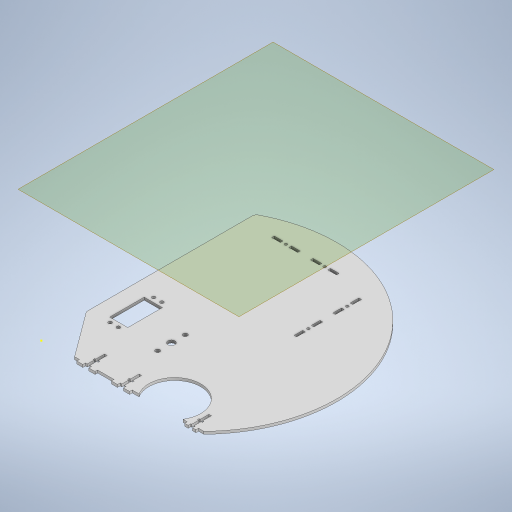
# Autodesk Inventor part: боковые стороны головы
Saved by Autodesk Inventor 2023.2 (Build 272271030, 271C)
## iProperties
Created: 2024-01-31
Part Number: боковые стороны головы
Material: Типовые
Document SubType Name: Modeling
Designer: I9232
Density: 1 g/cm^3
Appearance: По умолчанию
Mass: 147.227 g
Surface Area: 1032.77 cm^2
Volume: 147.227 cm^3
Author: I9232
Autodesk Inventor part; units mm, degrees
ref_plane "YZ Plane" through (0, 0, 0) normal (1, 0, 0) x (0, 1, 0)
ref_plane "XZ Plane" through (0, 0, 0) normal (0, 1, 0) x (-1, 0, 0)
ref_plane "XY Plane" through (0, 0, 0) normal (0, 0, 1) x (1, 0, 0)
sketch "Эскиз1" plane through (0, 0, 0) normal (0, 1, 0) x (-1, 0, 0)
  line L0 (-188.1037, -96.7538) -> (-38.405, -96.7538)
  line L1 (0, -148.7467) -> (0, -343.7987)
  line L2 (-38.405, -96.7538) -> (0, -148.7467)
  arc A0 (-188.1037, -96.7538) -> (0, -343.7987) centre (-75.4996, -206.1503) ccw
  point P0 (0, 0)
  point P1 (-169.7729, -152.9638)
  dimension "d66" = 96.7538
  dimension "d67" = 148.7467
  dimension "d68" = 126.452
  constraints: 6 end point, 2 point on circle, 1 centre point, 1 horizontal, 1 perpendicular, 1 point on line
  measures "d66" distance from line of L0 point (0, 0)
  measures "d67" distance of point (0, 0) L1.start
  measures "d68" angle of L0 L2
extrude "Выдавливание2" add sketch "Эскиз1" along normal blind 3
sketch "Эскиз3" plane through (0, 0, 0) normal (0, -1, 0) x (1, 0, 0)
  circle A0 centre (138.4507, -112.6325) radius 30
  line L0 (146.7814, -112.6325) -> (51.9196, -112.6325) construction
  point P0 (0, 0)
  constraints: 2 end point, 1 centre point, 1 horizontal, 1 point on line
extrude "Выдавливание3" cut sketch "Эскиз3" against normal through all
sketch "Эскиз4" plane through (0, 3, 0) normal (0, 1, 0) x (1, 0, 0)
  line L0 (40, 196.7538) -> (19, 196.7538)
  line L1 (19, 196.7538) -> (19, 156.7538)
  line L2 (19, 156.7538) -> (40, 156.7538)
  line L3 (40, 156.7538) -> (40, 196.7538)
  line L4 (40, 176.7538) -> (19, 176.7538) construction
  circle A0 centre (34.25, 201.9538) radius 1.95
  circle A1 centre (24.75, 201.9538) radius 1.95
  line L5 (0, 343.7987) -> (0, 148.7467) projected
  line L6 (29.5, 196.7538) -> (29.5, 203.7538) construction
  line L7 (39, 207.1538) -> (20, 207.1538) construction
  line L8 (39, 207.1538) -> (39, 196.7538) construction
  line L9 (20, 207.1538) -> (20, 196.7538) construction
  line L10 (34.25, 207.1538) -> (34.25, 196.7538) construction
  line L11 (24.75, 207.1538) -> (24.75, 196.7538) construction
  circle A2 centre (34.25, 151.5538) radius 1.95
  circle A3 centre (24.75, 151.5538) radius 1.95
  point P0 (0, 0)
  point P1 (39, 201.9538)
  dimension "d10" = 40
  dimension "d97" = 7
  dimension "d109" = 21
  dimension "d115" = 9.5
  dimension "d116" = 19
  dimension "d117" = 5.2
  dimension "d118" = 19
  dimension "d119" = 1
  dimension "d187" = 3.9
  constraints: 22 end point, 6 midpoint, 4 centre point, 4 point on line, 4 symmetric about line, 3 vertical, 2 parallel, 2 perpendicular, 1 equal radius, 1 horizontal, 2 other
  measures "d10" distance of L0.end L1.end
  measures "d97" distance of L6.start L6.end
  measures "d109" distance of L0.start L0.end
  measures "d115" distance of A1.centre A0.centre
  measures "d116" distance of L7.start L7.end
  measures "d117" distance from line of L0 A0.centre
  measures "d118" distance between parallel lines of L5 L1
  measures "d119" distance from line of L0.end L9
  measures "d187" diameter of A2
extrude "Выдавливание4" cut sketch "Эскиз4" against normal blind 10
sketch "Эскиз6" plane through (188.1037, 0, -96.7538) normal (0, 0, 1) x (1, 0, 0)
  line L0 (-24.1997, 3) -> (-75.1062, 3) construction
  line L1 (-83.1062, 3) -> (-90.1062, 3)
  line L2 (-90.1062, 3) -> (-90.1062, 0)
  line L3 (-90.1062, 0) -> (-83.1062, 0)
  line L4 (-83.1062, 0) -> (-83.1062, 3)
  line L5 (-97.1062, 3) -> (-104.1062, 3)
  line L6 (-104.1062, 3) -> (-104.1062, 0)
  line L7 (-104.1062, 0) -> (-97.1062, 0)
  line L8 (-97.1062, 0) -> (-97.1062, 3)
  line L9 (-123.1037, 3) -> (-130.1037, 3)
  line L10 (-130.1037, 3) -> (-130.1037, 0)
  line L11 (-130.1037, 0) -> (-123.1037, 0)
  line L12 (-123.1037, 0) -> (-123.1037, 3)
  line L13 (-137.1037, 3) -> (-144.1037, 3)
  line L14 (-144.1037, 3) -> (-144.1037, 0)
  line L15 (-144.1037, 0) -> (-137.1037, 0)
  line L16 (-137.1037, 0) -> (-137.1037, 3)
  line L17 (-188.1037, 0) -> (-75.1062, 0)
  line L18 (0, 0) -> (0, 3)
  line L19 (-188.1037, 0) -> (-188.1037, 3) construction
  line L20 (-6.1997, 3) -> (-10.1997, 3)
  line L21 (-10.1997, 3) -> (-10.1997, 0)
  line L22 (-10.1997, 0) -> (-6.1997, 0)
  line L23 (-6.1997, 0) -> (-6.1997, 3)
  line L24 (-15.1997, 3) -> (-19.1997, 3)
  line L25 (-19.1997, 3) -> (-19.1997, 0)
  line L26 (-19.1997, 0) -> (-15.1997, 0)
  line L27 (-15.1997, 0) -> (-15.1997, 3)
  line L28 (-24.1997, 3) -> (0, 3) construction
  line L29 (-24.1997, 3) -> (-24.1997, 0)
  line L30 (-75.1062, 0) -> (-75.1062, 3) construction
  point P0 (-97.1062, 1.5)
  point P1 (-90.1062, 1.5)
  point P2 (-137.1037, 1.5)
  point P3 (-130.1037, 1.5)
  point P4 (-126.6037, 0)
  point P5 (-140.6037, 0)
  point P6 (-188.1037, 1.5)
  point P7 (-15.1997, 1.5)
  point P8 (-10.1997, 1.5)
  point P9 (-75.1062, 1.5)
  point P10 (-83.1062, 1.5)
  dimension "d26" = 3
  dimension "d91" = 8
  constraints: 62 end point, 13 parallel, 11 midpoint, 6 horizontal, 6 perpendicular, 4 point on line
  measures "d26" distance of L15.end L13.start
  measures "d91" distance of point (-75.106, 1.5) point (-83.106, 1.5)
sketch "Эскиз7" plane through (0, 0, 0) normal (0, -1, 0) x (1, 0, 0)
  line L0 (54.5455, -116.7538) -> (54.5455, -96.7267) construction
  line L1 (51.95, -104.8537) -> (51.95, -106.6537)
  line L2 (57.55, -106.6537) -> (57.55, -104.8537)
  line L3 (57.55, -104.8537) -> (51.95, -106.6537) construction
  line L4 (51.95, -104.8537) -> (57.55, -106.6537) construction
  line L5 (57.55, -104.8537) -> (55.9955, -104.8537)
  line L6 (53.0955, -104.8537) -> (51.95, -104.8537)
  line L7 (51.95, -106.6537) -> (53.0955, -106.6537)
  line L8 (55.9955, -106.6537) -> (57.55, -106.6537)
  line L9 (55.9955, -96.7538) -> (55.9955, -104.8537)
  line L10 (55.9955, -106.6537) -> (55.9955, -116.755)
  line L11 (53.0955, -96.7538) -> (53.0955, -104.8537)
  line L12 (53.0955, -106.6537) -> (53.0955, -116.755)
  line L13 (91.7425, -104.8538) -> (91.7425, -106.6538)
  line L14 (97.3425, -106.6538) -> (97.3425, -104.8538)
  line L15 (97.3425, -104.8538) -> (91.7425, -106.6538) construction
  line L16 (91.7425, -104.8538) -> (97.3425, -106.6538) construction
  line L17 (97.3425, -104.8538) -> (95.9925, -104.8538)
  line L18 (93.0925, -104.8538) -> (91.7425, -104.8538)
  line L19 (91.7425, -106.6538) -> (93.0925, -106.6538)
  line L20 (95.9925, -106.6538) -> (97.3425, -106.6538)
  line L21 (95.9925, -96.6922) -> (95.9925, -104.8538)
  line L22 (95.9925, -106.6538) -> (95.9925, -116.6921)
  line L23 (93.0925, -96.6922) -> (93.0925, -104.8538)
  line L24 (93.0925, -106.6538) -> (93.0925, -116.6921)
  line L25 (172.6039, -104.8538) -> (172.6039, -106.6538)
  line L26 (178.2039, -106.6538) -> (178.2039, -104.8538)
  line L27 (178.2039, -104.8538) -> (172.6039, -106.6538) construction
  line L28 (172.6039, -104.8538) -> (178.2039, -106.6538) construction
  line L29 (178.2039, -104.8538) -> (176.8539, -104.8538)
  line L30 (173.9539, -104.8538) -> (172.6039, -104.8538)
  line L31 (172.6039, -106.6538) -> (173.9539, -106.6538)
  line L32 (176.8539, -106.6538) -> (178.2039, -106.6538)
  line L33 (176.8539, -96.7538) -> (176.8539, -104.8538)
  line L34 (176.8539, -106.6538) -> (176.8539, -116.7538)
  line L35 (173.9539, -96.7538) -> (173.9539, -104.8538)
  line L36 (173.9539, -106.6538) -> (173.9539, -116.7538)
  line L37 (95.9925, -116.6921) -> (93.0925, -116.6921)
  line L38 (95.9925, -96.6922) -> (93.0925, -96.6922) construction
  line L39 (38.405, -96.7538) -> (112.9975, -96.7538) projected
  line L40 (0, -343.7987) -> (0, -148.7467) projected
  line L41 (176.8539, -96.7538) -> (173.9539, -96.7538)
  line L42 (163.9039, -96.7538) -> (188.1037, -96.7538)
  line L43 (176.9039, -96.7538) -> (173.9039, -96.7538) projected
  line L44 (176.8539, -116.7538) -> (173.9539, -116.7538)
  line L45 (55.9955, -116.755) -> (53.0955, -116.755)
  point P0 (0, 0)
  point P1 (94.5425, -96.6922)
  point P2 (75.7012, -96.7538)
  point P3 (95.9925, -96.7538)
  point P4 (93.0925, -96.7538)
  point P5 (175.4039, -96.7538)
  point P6 (172.6039, -105.7538)
  point P7 (96.6675, -104.8538)
  point P8 (55.9955, -100.8037)
  point P9 (55.9955, -96.7538)
  point P10 (53.0955, -96.7538)
  dimension "d140" = 5.6
  dimension "d164" = 39.997
  dimension "d172" = 2.9
  dimension "d174" = 8.1
  dimension "d176" = 5.6
  dimension "d177" = 2.9
  dimension "d178" = 5.6
  dimension "d179" = 1.8
  dimension "d180" = 8.1
  dimension "d181" = 1.8
  dimension "d182" = 2.9
  dimension "d183" = 2.9
  dimension "d186" = 1.8
  constraints: 86 end point, 17 parallel, 14 equal length, 13 perpendicular, 10 horizontal, 6 midpoint, 2 point on line, 2 symmetric about line, 1 vertical, 2 other
  measures "d140" distance between parallel lines of L1 L2
  measures "d164" distance of point (94.542, -96.692) L0.end
  measures "d172" distance of L34.end L36.end
  measures "d174" distance of L33.start L33.end
  measures "d176" distance from line of point (172.604, -105.754) L26
  measures "d177" distance of L22.end L24.end
  measures "d178" distance between parallel lines of L13 L14
  measures "d179" distance of L14.start L14.end
  measures "d181" distance of L2.start L2.end
  measures "d182" distance of L10.end L45.end
  measures "d183" distance from line of L11 point (55.995, -100.804)
  measures "d186" distance of L26.start L26.end
extrude "Выдавливание6" cut sketch "Эскиз7" against normal blind 3
sketch "Эскиз10" plane through (0, 0, 0) normal (0, -1, 0) x (1, 0, 0)
  line L0 (147.1367, -255.2231) -> (147.1367, -245.2231)
  line L1 (144.1393, -255.2231) -> (147.1367, -255.2231)
  line L2 (144.1393, -245.2231) -> (144.1393, -255.2231)
  line L3 (147.1367, -245.2231) -> (144.1393, -245.2231)
  line L4 (147.1367, -265.2231) -> (144.1393, -265.2231)
  line L5 (147.1367, -275.2231) -> (147.1367, -265.2231)
  line L6 (144.1393, -265.2231) -> (144.1393, -275.2231)
  line L7 (144.1393, -275.2231) -> (147.1367, -275.2231)
  line L8 (147.1367, -290.2231) -> (144.1393, -290.2231)
  line L9 (147.1367, -300.2231) -> (147.1367, -290.2231)
  line L10 (144.1393, -300.2231) -> (147.1367, -300.2231)
  line L11 (144.1393, -290.2231) -> (144.1393, -300.2231)
  line L12 (147.1367, -310.2231) -> (144.1393, -310.2231)
  line L13 (147.1367, -320.2231) -> (147.1367, -310.2231)
  line L14 (144.1393, -320.2231) -> (147.1367, -320.2231)
  line L15 (144.1393, -310.2231) -> (144.1393, -320.2231)
  line L16 (145.638, -255.2231) -> (145.638, -265.2231) construction
  circle A0 centre (145.638, -260.2231) radius 1.5
  circle A1 centre (145.638, -305.2231) radius 1.5
  line L17 (145.638, -300.2231) -> (145.638, -310.2231) construction
  point P0 (0, 0)
  dimension "d184" = 3
  constraints: 36 end point, 6 midpoint, 2 centre point, 1 equal radius
  measures "d184" diameter of A0
extrude "Выдавливание8" cut sketch "Эскиз10" against normal blind 3
sketch "Эскиз11" plane through (0, 0, 0) normal (0, -1, 0) x (1, 0, 0)
  circle A0 centre (80.5, -166.7538) radius 4
  line L0 (0, -343.7987) -> (0, -148.7467) projected
  line L1 (38.405, -96.7538) -> (112.9975, -96.7538) projected
  point P0 (0, 0)
  point P1 (65, -96.7538)
  point P2 (83.9975, -96.7538)
  dimension "d130" = 80.5
  dimension "d131" = 70
  dimension "d132" = 8
  constraints: 1 centre point
  measures "d130" distance from line of L0 A0.centre
  measures "d131" distance from line of L1 A0.centre
  measures "d132" diameter of A0
extrude "Выдавливание9" cut sketch "Эскиз11" against normal blind 3
ref_plane "РабПлоскость3" through (116.247, 153.6358, -229.9493) normal (0, -1, 0) x (-1, 0, 0)
sketch "Эскиз14" plane through (0, 3, 0) normal (0, 1, 0) x (1, 0, 0)
  line L0 (97.9377, 333.374) -> (107.9377, 333.374)
  line L1 (107.9377, 333.374) -> (107.9377, 330.3766)
  line L2 (97.9377, 330.3766) -> (97.9377, 333.374)
  line L3 (107.9377, 330.3766) -> (97.9377, 330.3766)
  line L4 (77.9377, 333.374) -> (77.9377, 330.374)
  line L5 (77.9377, 330.374) -> (87.9377, 330.374)
  line L6 (87.9377, 330.374) -> (87.9377, 333.374)
  line L7 (87.9377, 333.374) -> (77.9377, 333.374)
  line L8 (52.9377, 333.374) -> (52.9377, 330.374)
  line L9 (52.9377, 330.374) -> (62.9377, 330.374)
  line L10 (62.9377, 330.374) -> (62.9377, 333.374)
  line L11 (62.9377, 333.374) -> (52.9377, 333.374)
  line L12 (32.9377, 333.374) -> (32.9377, 330.374)
  line L13 (32.9377, 330.374) -> (42.9377, 330.374)
  line L14 (42.9377, 330.374) -> (42.9377, 333.374)
  line L15 (42.9377, 333.374) -> (32.9377, 333.374)
  circle A0 centre (92.9377, 331.8747) radius 1.5
  circle A1 centre (47.9377, 331.874) radius 1.5
  line L16 (87.9377, 331.874) -> (97.9377, 331.8753)
  line L17 (52.9377, 331.874) -> (42.9377, 331.874)
  point P0 (0, 0)
  dimension "d127" = 3
  constraints: 36 end point, 6 midpoint, 2 centre point, 1 equal radius, 1 other
  measures "d127" diameter of A0
extrude "Выдавливание10" cut sketch "Эскиз14" against normal up to surface (3 mm away)
extrude "Выдавливание11" add sketch "Эскиз6" along normal blind 3
sketch "Эскиз15" plane through (172.9039, 0, -96.7538) normal (0, 0, 1) x (1, 0, 0)
  point P0 (-172.9039, 0)
sketch "Эскиз16" plane through (0, 0, 0) normal (0, -1, 0) x (1, 0, 0)
  circle A0 centre (80.5, -182.7538) radius 2.5
  circle A1 centre (80.5, -150.7538) radius 2.5
  circle A2 centre (80.5, -166.7538) radius 4 construction
  line L0 (80.5, -150.7538) -> (80.5, -182.7538) construction
  point P0 (0, 0)
  point P1 (80.5, -166.7538)
  dimension "d188" = 5
  dimension "d189" = 32
  constraints: 2 centre point, 2 end point, 1 coincident, 1 equal radius, 1 midpoint, 1 vertical
  measures "d188" diameter of A1
  measures "d189" distance of L0.start L0.end
extrude "Выдавливание12" cut sketch "Эскиз16" against normal blind 3
fillet "Сопряжение1" radius 5 2 edges at (0, 1.5, -343.7987) (0, 1.5, -148.7467)
